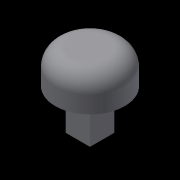
# Autodesk Inventor part: power button
Saved by Autodesk Inventor 2014 (Build 180170000, 170)
## iProperties
Created: 2014-11-06
Part Number: power button
Material: Generic
Document SubType Name: Modeling
Designer: Scott
Density: 1 g/cm^3
Appearance: Default
Author: Scott
Autodesk Inventor part; units mm, degrees
ref_plane "YZ Plane" through (0, 0, 0) normal (1, 0, 0) x (0, 1, 0)
ref_plane "XZ Plane" through (0, 0, 0) normal (0, 1, 0) x (-1, 0, 0)
ref_plane "XY Plane" through (0, 0, 0) normal (0, 0, 1) x (1, 0, 0)
sketch "Sketch1" plane through (0, 0, 0) normal (0, 1, 0) x (-1, 0, 0)
  line L0 (0, 0) -> (3.302, 0)
  line L1 (3.302, 0) -> (3.302, 3.302)
  line L2 (3.302, 3.302) -> (0, 3.302)
  line L3 (0, 3.302) -> (0, 0)
  line L4 (3.9389, 3.9389) -> (3.9389, -0.6369)
  line L5 (3.9389, -0.6369) -> (-0.6369, -0.6369)
  line L6 (-0.6369, -0.6369) -> (-0.6369, 3.9389)
  line L7 (-0.6369, 3.9389) -> (3.9389, 3.9389)
  dimension "d0" = 3.302
  dimension "d1" = 3.302
  constraints: 16 end point, 4 parallel, 2 perpendicular, 1 horizontal, 3 other
  measures "d0" distance of L0.start L0.end
  measures "d1" distance of L0.end L1.end
extrude "Extrusion1" add sketch "Sketch1" along normal blind 7.62
sketch "Sketch2" plane through (0, 7.62, 0) normal (0, 1, 0) x (1, 0, 0)
  circle A0 centre (-1.651, -1.651) radius 6.535
  constraints: 1 centre point
extrude "Extrusion2" add sketch "Sketch2" along normal blind 6.35
fillet "Fillet1" radius 3.175 1 edges at (-8.186, 13.97, 1.651)
body "Solid1"
